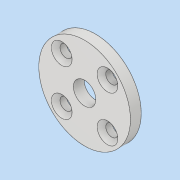
# Autodesk Inventor part: idlerShaftBearingMount
Saved by Autodesk Inventor 2017 (Build 210142000, 142)
## iProperties
Created: 2016-11-30
Part Number: idlerShaftBearingMount
Material: ABS Plastic
Document SubType Name: Modeling
Designer: techn
Density: 1.06 g/cm^3
Appearance: Smooth - White
Author: techn
Autodesk Inventor part; units mm, degrees
ref_plane "YZ Plane" through (0, 0, 0) normal (1, 0, 0) x (0, 1, 0)
ref_plane "XZ Plane" through (0, 0, 0) normal (0, 1, 0) x (-1, 0, 0)
ref_plane "XY Plane" through (0, 0, 0) normal (0, 0, 1) x (1, 0, 0)
sketch "Sketch1" plane through (0, 0, 0) normal (0, 0, 1) x (1, 0, 0)
  line L0 (0, 0) -> (6.7352, 6.7352)
  line L1 (0, 0) -> (9.525, 0) construction
  circle A0 centre (6.7352, 6.7352) radius 1.778
  circle A1 centre (-6.7352, 6.7352) radius 1.778
  circle A2 centre (-6.7352, -6.7352) radius 1.778
  circle A3 centre (6.7352, -6.7352) radius 1.778
  circle A4 centre (0, 0) radius 13.4938
  circle A5 centre (0, 0) radius 3.302
  dimension "d0" = 9.525
  dimension "d1" = 45
  dimension "d2" = 3.556
  dimension "d5" = 360
  dimension "d7" = 26.9875
  dimension "d8" = 6.604
  constraints: 6 centre point, 4 end point, 3 coincident, 1 equal length, 1 horizontal, 9 other
  measures "d0" distance of L0.start L0.end
  measures "d1" angle of L1 L0
  measures "d2" diameter of A0
  measures "d7" diameter of A4
  measures "d8" diameter of A5
extrude "Extrusion1" add sketch "Sketch1" along normal blind 3.175
chamfer "Chamfer1" distance 1.27 angle 45 4 edges at (-8.5132, 6.7352, 3.175) (4.9572, 6.7352, 3.175) (4.9572, -6.7352, 3.175) (-8.5132, -6.7352, 3.175)
body "Solid1"
